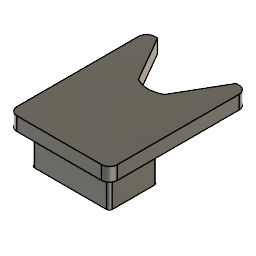
workout-dumbbell-holder (Autodesk Fusion 360 design; units mm, degrees)
Autodesk Fusion 360 part; units mm, degrees
ref_plane "WorkPlane3" through (0, 0, -38) normal (0, 0, 1) x (1, 0, 0)
sketch "Sketch6" plane through (0, 0, -38) normal (0, 0, 1) x (1, 0, 0)
  line L0 (-34.25, -21.25) -> (34.25, -21.25)
  line L1 (34.25, -21.25) -> (34.25, 21.25)
  line L2 (34.25, 21.25) -> (-34.25, 21.25)
  line L3 (-34.25, 21.25) -> (-34.25, -21.25)
extrude "Extrude6" add sketch "Sketch6" along normal blind 30
fillet "Fillet7" radius 2.5 4 edges at (-34.25, 21.25, -23) (34.25, 21.25, -23) (34.25, -21.25, -23) (-34.25, -21.25, -23)
ref_plane "WorkPlane4" through (0, 0, -8) normal (0, 0, 1) x (1, 0, 0)
sketch "Sketch7" plane through (0, 0, -8) normal (0, 0, 1) x (1, 0, 0)
  line L0 (-44.25, -31.25) -> (44.25, -31.25)
  line L1 (44.25, -31.25) -> (44.25, 90)
  line L2 (44.25, 90) -> (-44.25, 90)
  line L3 (-44.25, 90) -> (-44.25, -31.25)
extrude "Extrude7" add sketch "Sketch7" along normal blind 12
fillet "Fillet8" radius 7 4 edges at (-44.25, 90, -2) (44.25, 90, -2) (44.25, -31.25, -2) (-44.25, -31.25, -2)
sketch "Sketch8" plane through (0, 0, -8) normal (0, 0, 1) x (1, 0, 0)
  line L0 (-34.547, 90) -> (-11.5, 50.0814)
  arc A0 (-11.5, 50.0814) -> (11.5, 50.0814) centre (0, 70) ccw
  line L1 (11.5, 50.0814) -> (34.547, 90)
  line L2 (34.547, 90) -> (34.547, 95)
  line L3 (34.547, 95) -> (-34.547, 95)
  line L4 (-34.547, 95) -> (-34.547, 90)
extrude "Extrude8" cut sketch "Sketch8" along normal blind 12
fillet "Fillet9" radius 5 64 edges at (33.5178, -20.5178, -8) (0, -21.25, -8) (-33.5178, -20.5178, -8) (-34.25, 0, -8) (-33.5178, 20.5178, -8) (0, 21.25, -8) (33.5178, 20.5178, -8) (34.25, 0, -8) (34.25, 0, -8) (33.5178, 20.5178, -8) (0, 21.25, -8) (-33.5178, 20.5178, -8) (-34.25, 0, -8) (-33.5178, -20.5178, -8) (0, -21.25, -8) (33.5178, -20.5178, -8) (33.5178, 20.5178, -8) (34.25, 0, -8) (33.5178, -20.5178, -8) (0, -21.25, -8) (-33.5178, -20.5178, -8) (-34.25, 0, -8) (-33.5178, 20.5178, -8) (0, 21.25, -8) (0, 21.25, -8) (-33.5178, 20.5178, -8) (-34.25, 0, -8) (-33.5178, -20.5178, -8) (0, -21.25, -8) (33.5178, -20.5178, -8) (34.25, 0, -8) (33.5178, 20.5178, -8) (-33.5178, 20.5178, -8) (0, 21.25, -8) (33.5178, 20.5178, -8) (34.25, 0, -8) (33.5178, -20.5178, -8) (0, -21.25, -8) (-33.5178, -20.5178, -8) (-34.25, 0, -8) (-34.25, 0, -8) (-33.5178, -20.5178, -8) (0, -21.25, -8) (33.5178, -20.5178, -8) (34.25, 0, -8) (33.5178, 20.5178, -8) (0, 21.25, -8) (-33.5178, 20.5178, -8) (-33.5178, -20.5178, -8) (-34.25, 0, -8) (-33.5178, 20.5178, -8) (0, 21.25, -8) (33.5178, 20.5178, -8) (34.25, 0, -8) (33.5178, -20.5178, -8) (0, -21.25, -8) (0, -21.25, -8) (33.5178, -20.5178, -8) (34.25, 0, -8) (33.5178, 20.5178, -8) (0, 21.25, -8) (-33.5178, 20.5178, -8) (-34.25, 0, -8) (-33.5178, -20.5178, -8)
named bodies: "holder"
